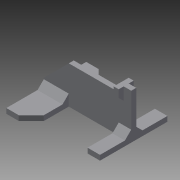
# Autodesk Inventor part: Pata
Saved by Autodesk Inventor 2014 SP1 (Build 180222100, 222)
## iProperties
Created: 2013-11-10
Part Number: Pata
Material: Genérico
Document SubType Name: Modeling
Designer: Gregorio
Density: 1 g/cm^3
Appearance: Valor por defecto
Author: Gregorio
Autodesk Inventor part; units mm, degrees
ref_plane "YZ Plane" through (0, 0, 0) normal (1, 0, 0) x (0, 1, 0)
ref_plane "XZ Plane" through (0, 0, 0) normal (0, 1, 0) x (-1, 0, 0)
ref_plane "XY Plane" through (0, 0, 0) normal (0, 0, 1) x (1, 0, 0)
sketch "Boceto1" plane through (0, 0, 0) normal (0, 1, 0) x (-1, 0, 0)
  line L0 (0, 0) -> (70, 0)
  line L1 (70, 0) -> (70, 30)
  line L2 (70, 30) -> (0, 30)
  line L3 (0, 30) -> (0, 0)
  line L4 (0, 30) -> (10, 30)
  line L5 (10, 30) -> (10, 36)
  line L6 (10, 36) -> (0, 36)
  line L7 (0, 36) -> (0, 30)
  dimension "d0" = 10
  dimension "d14" = 70
  constraints: 16 end point, 4 parallel, 2 horizontal, 2 perpendicular
  measures "d0" distance of L6.end L5.end
  measures "d14" distance of L0.start L0.end
extrude "Extrusión1" add sketch "Boceto1" along normal blind 4
sketch "Boceto2" plane through (0, 4, 0) normal (0, 1, 0) x (1, 0, 0)
  line L0 (-10, -30) -> (-6, -30)
  line L1 (-6, -30) -> (-6, -36)
  line L2 (-6, -36) -> (-10, -36)
  line L3 (-10, -36) -> (-10, -30)
  constraints: 8 end point, 2 parallel, 1 horizontal, 1 perpendicular
extrude "Extrusión2" add sketch "Boceto2" along normal blind 4
chamfer "Chaflán1" distance 20 angle 45 1 edges at (-70, 2, 30)
sketch "Boceto6" plane through (0, 4, 0) normal (0, 1, 0) x (1, 0, 0)
  line L0 (-70, 0) -> (-50, 0)
  line L1 (-50, 0) -> (-50, -4)
  line L2 (-50, -4) -> (-70, -4)
  line L3 (-70, -4) -> (-70, 0)
  dimension "d15" = 20
  constraints: 8 end point, 2 parallel, 1 horizontal, 1 perpendicular
  measures "d15" distance of L0.start L0.end
extrude "Extrusión4" add sketch "Boceto6" along normal blind 30
chamfer "Chaflán2" distance 10 angle 45 1 edges at (-50, 34, 2)
sketch "Boceto7" plane through (0, 0, 0) normal (0, -1, 0) x (1, 0, 0)
  line L0 (-70, 0) -> (-50, 0)
  line L1 (-50, 0) -> (-50, 4)
  line L2 (-50, 4) -> (-70, 4)
  line L3 (-70, 4) -> (-70, 0)
  dimension "d19" = 20
  constraints: 8 end point, 2 parallel, 1 horizontal, 1 perpendicular
  measures "d19" distance of L2.end L1.end
extrude "Extrusión5" add sketch "Boceto7" along normal blind 30
sketch "Boceto8" plane through (0, 0, 0) normal (0, -1, 0) x (1, 0, 0)
  line L0 (-10, 36) -> (0, 36) projected
  line L1 (-10, 30) -> (-6, 30)
  line L2 (-6, 30) -> (-6, 36)
  line L3 (-6, 36) -> (-10, 36)
  line L4 (-10, 36) -> (-10, 30)
  constraints: 8 end point, 2 parallel, 1 horizontal, 1 perpendicular, 1 point on line
extrude "Extrusión6" add sketch "Boceto8" along normal blind 4
chamfer "Chaflán3" distance 10 angle 45 1 edges at (-50, -30, 2)
sketch "Boceto9" plane through (0, 0, 0) normal (0, -1, 0) x (1, 0, 0)
  line L0 (0, 36) -> (0, 0) projected
  line L1 (0, 0) -> (0, 4)
  line L2 (0, 4) -> (-10, 4)
  line L3 (-10, 4) -> (-10, 0)
  line L4 (-10, 0) -> (0, 0)
  constraints: 8 end point, 2 parallel, 1 perpendicular, 1 point on line
extrude "Extrusión7" add sketch "Boceto9" along normal blind 25
sketch "Boceto10" plane through (0, 4, 0) normal (0, 1, 0) x (1, 0, 0)
  line L0 (0, -36) -> (0, 0) projected
  line L1 (0, 0) -> (0, -4)
  line L2 (0, -4) -> (-10, -4)
  line L3 (-10, -4) -> (-10, 0)
  line L4 (-10, 0) -> (0, 0)
  constraints: 8 end point, 2 parallel, 1 perpendicular, 1 point on line
extrude "Extrusión8" add sketch "Boceto10" along normal blind 25
chamfer "Chaflán4" distance 5 angle 45 4 edges at (-60, 0, 4) (-5, 0, 4) (-60, 4, 4) (-5, 4, 4)
chamfer "Chaflán5" distance 4 angle 45 2 edges at (-8, 4, 30) (-8, 0, 30)
